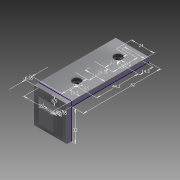
# Autodesk Inventor part: keithley_2000_front_feet
Saved by Autodesk Inventor 2015 (Build 190159000, 159)
## iProperties
Created: 2015-05-21
Part Number: keithley_2000_front_feet
Material: Generic
Document SubType Name: Modeling
Designer: Justin
Density: 1 g/cm^3
Appearance: Default
Author: Justin
Autodesk Inventor part; units mm, degrees
ref_plane "YZ Plane" through (0, 0, 0) normal (1, 0, 0) x (0, 1, 0)
ref_plane "XZ Plane" through (0, 0, 0) normal (0, 1, 0) x (-1, 0, 0)
ref_plane "XY Plane" through (0, 0, 0) normal (0, 0, 1) x (1, 0, 0)
sketch "Sketch1" plane through (0, 0, 0) normal (0, 0, 1) x (1, 0, 0)
  line L0 (0, 0) -> (35, 0)
  line L1 (35, 0) -> (35, 82)
  line L2 (35, 82) -> (0, 82)
  line L3 (0, 82) -> (0, 0)
  line L4 (8.5, 79.95) -> (8.5, 77.05)
  line L5 (8.5, 77.05) -> (5.5, 77.05)
  line L6 (5.5, 77.05) -> (5.5, 53.95)
  line L7 (5.5, 33.6) -> (5.5, 6.85)
  line L8 (5.5, 6.85) -> (29.5, 6.85)
  line L9 (29.5, 6.85) -> (29.5, 79.95)
  line L10 (29.5, 79.95) -> (8.5, 79.95)
  line L11 (5.5, 53.95) -> (8.5, 53.95)
  line L12 (8.5, 53.95) -> (8.5, 33.6)
  line L13 (8.5, 33.6) -> (5.5, 33.6)
  circle A0 centre (19, 65.65) radius 2.25
  circle A1 centre (19, 21.45) radius 2.25
  dimension "d0" = 35
  dimension "d1" = 82
  dimension "d2" = 21
  dimension "d3" = 24
  dimension "d4" = 21
  dimension "d5" = 26.75
  dimension "d6" = 23.1
  dimension "d7" = 26
  dimension "d8" = 6.85
  dimension "d9" = 5.5
  dimension "d10" = 20.35
  dimension "d15" = 4.5
  dimension "d16" = 4.5
  dimension "d17" = 44.2
  dimension "d18" = 10.5
  dimension "d19" = 14.3
  dimension "d20" = 10.5
  constraints: 28 end point, 8 perpendicular, 2 centre point, 2 horizontal, 2 parallel, 2 point on line, 1 vertical
  measures "d0" distance of L0.start L0.end
  measures "d1" distance of L0.end L1.end
  measures "d2" distance of L9.end L4.start
  measures "d3" distance between parallel lines of L9 L6
  measures "d4" distance between parallel lines of L9 L12
  measures "d5" distance of L7.start L7.end
  measures "d6" distance of L5.end L6.end
  measures "d7" distance between parallel lines of L11 L10
  measures "d8" distance between parallel lines of L0 L8
  measures "d9" distance between parallel lines of L1 L9
  measures "d10" distance of L11.end L12.end
  measures "d15" diameter of A1
  measures "d16" diameter of A0
  measures "d17" distance of A0.centre A1.centre
  measures "d18" distance from line of L9 A0.centre
  measures "d19" distance from line of L10 A0.centre
  measures "d20" distance from line of L9 A1.centre
extrude "Extrusion1" add sketch "Sketch1" against normal blind 1.5 contours L10 L9 L8 L7 L13 L12 L11 L6 L5 L4 | A0 | A1
extrude "Extrusion3" add sketch "Sketch1" along normal blind 5 contours L3 L2 L1 L0 | L10 L9 L8 L7 L13 L12 L11 L6 L5 L4
sketch "Sketch2" plane through (0, 0, 5) normal (0, 0, 1) x (1, 0, 0)
  circle A0 centre (19, 21.45) radius 4.25
  circle A1 centre (19, 65.65) radius 4.25
  point P0 (0, 0)
  dimension "d23" = 8.5
  dimension "d24" = 8.5
  constraints: 2 centre point, 2 coincident
  measures "d23" diameter of A0
  measures "d24" diameter of A1
extrude "Extrusion4" cut sketch "Sketch2" against normal blind 3
sketch "Sketch3" plane through (0, 0, 0) normal (0, -1, 0) x (1, 0, 0)
  line L0 (0, 5) -> (35, 5) projected
  line L1 (0, 0) -> (0, 5) projected
  line L2 (35, 0) -> (35, 5) projected
  line L3 (0, 5) -> (35, 5)
  line L4 (35, 5) -> (35, -32)
  line L5 (35, -32) -> (0, -32)
  line L6 (0, -32) -> (0, 5)
  line L7 (0, 0) -> (35, 0) projected
  line L8 (5.5, 0) -> (5.5, -1.5) projected
  line L9 (5.5, -8.5) -> (24.15, -8.5)
  line L10 (24.15, -8.5) -> (24.15, -11.35)
  line L11 (24.15, -11.35) -> (5.5, -11.35)
  line L12 (5.5, -11.35) -> (5.5, -8.5)
  dimension "d27" = 32
  dimension "d28" = 8.5
  dimension "d29" = 2.85
  dimension "d30" = 18.65
  constraints: 16 end point, 4 parallel, 2 collinear, 2 horizontal, 2 perpendicular
  measures "d27" distance between parallel lines of L5 L7
  measures "d28" distance between parallel lines of L9 L7
  measures "d29" distance of L9.end L10.end
  measures "d30" distance of L10.end L11.end
extrude "Extrusion5" add sketch "Sketch3" along normal blind 5 contours L0 L2 L7 L1 | L7 L4 L5 L6 | L9 L10 L11 L12
extrude "Extrusion6" add sketch "Sketch3" against normal blind 1.5 contours L9 L10 L11 L12
fillet "Fillet1" radius 1 1 edges at (29.5, 79.95, -0.75)
fillet "Fillet2" radius 1 1 edges at (8.5, 79.95, -0.75)
fillet "Fillet3" radius 1 1 edges at (5.5, 77.05, -0.75)
fillet "Fillet4" radius 1 1 edges at (5.5, 53.95, -0.75)
fillet "Fillet5" radius 1 1 edges at (5.5, 33.6, -0.75)
fillet "Fillet6" radius 1 1 edges at (5.5, 6.85, -0.75)
fillet "Fillet7" radius 1 1 edges at (29.5, 6.85, -0.75)
fillet "Fillet8" radius 1 1 edges at (5.5, 0.75, -11.35)
fillet "Fillet9" radius 1 3 edges at (24.15, 0.75, -11.35) (24.15, 0.75, -8.5) (5.5, 0.75, -8.5)
extrude "Extrusion7" cut sketch "Sketch1" against normal up to next contours A0 | A1
sketch "Sketch4" plane through (0, -5, 0) normal (0, -1, 0) x (1, 0, 0)
  line L0 (25.5, -24) -> (9.5, -24)
  line L1 (9.5, -24) -> (9.5, -8)
  line L2 (9.5, -8) -> (25.5, -8)
  line L3 (25.5, -8) -> (25.5, -24)
  line L4 (0, 5) -> (0, -32) projected
  line L5 (0, -32) -> (35, -32) projected
  point P0 (0, 0)
  dimension "d46" = 16
  dimension "d47" = 16
  dimension "d48" = 9.5
  dimension "d49" = 8
  constraints: 8 end point, 2 parallel, 1 horizontal, 1 perpendicular
  measures "d46" distance of L0.start L0.end
  measures "d47" distance of L0.end L1.end
  measures "d48" distance between parallel lines of L4 L1
  measures "d49" distance between parallel lines of L5 L0
extrude "Extrusion8" add sketch "Sketch4" along normal blind 5
chamfer "Chamfer1" distance 5 angle 45 4 edges at (9.5, -5, -16) (17.5, -5, -24) (25.5, -5, -16) (17.5, -5, -8)
body "Solid1"
